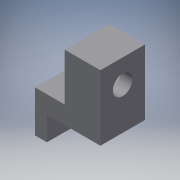
# Autodesk Inventor part: TMP_Holder_MTP
Saved by Autodesk Inventor 2019.4 (Build 234330000, 330)
## iProperties
Created: 2021-04-17
Part Number: TMP_Holder_MTP
Material: Generic
Document SubType Name: Modeling
Designer: diederichbenedict
Density: 1 g/cm^3
Appearance: Default
Author: diederichbenedict
Autodesk Inventor part; units mm, degrees
ref_plane "YZ Plane" through (0, 0, 0) normal (1, 0, 0) x (0, 1, 0)
ref_plane "XZ Plane" through (0, 0, 0) normal (0, 1, 0) x (-1, 0, 0)
ref_plane "XY Plane" through (0, 0, 0) normal (0, 0, 1) x (1, 0, 0)
sketch "Sketch1" plane through (0, 0, 0) normal (0, 0, 1) x (1, 0, 0)
  line L0 (31.7273, 1.5) -> (12.134, 1.5)
  line L1 (31.7273, -1.5) -> (12.134, -1.5)
  line L2 (16.2594, -4) -> (22.2594, -4)
  line L3 (22.2594, -4) -> (22.2594, 4)
  line L4 (22.2594, 4) -> (16.2594, 4)
  line L5 (16.2594, 4) -> (16.2594, -4)
  line L6 (16.2594, -4) -> (22.2594, 4) construction
  line L7 (22.2594, -4) -> (16.2594, 4) construction
  point P0 (0, 0)
  point P1 (19.2594, 0)
  dimension "d0" = 8
  dimension "d1" = 6
  constraints: 16 end point, 3 horizontal, 2 midpoint, 2 parallel, 1 perpendicular, 4 other
  measures "d0" distance between parallel lines of L2 L4
  measures "d1" distance between parallel lines of L3 L5
extrude "Extrusion1" add sketch "Sketch1" along normal mid plane 7.5
sketch "Sketch2" plane through (16.2594, -4, 3.75) normal (-1, 0, 0) x (0, 0, 1)
  line L0 (0, 0) -> (-7.5, 0) projected
  line L1 (0, 8) -> (0, 0) projected
  line L2 (-7.5, 8) -> (0, 8) projected
  line L3 (-7.5, 0) -> (-7.5, 8) projected
  circle A0 centre (-3.75, 4) radius 1.65
  dimension "d17" = 3.3
  constraints: 1 centre point
  measures "d17" diameter of A0
extrude "Extrusion2" cut sketch "Sketch2" against normal through all contours A0
sketch "Sketch3" plane through (16.2594, -4, 3.75) normal (-1, 0, 0) x (0, 0, 1)
  point P0 (-3.75, 4)
sketch "Sketch4" plane through (16.2594, -4, 3.75) normal (-1, 0, 0) x (0, 0, 1)
  line L0 (-0.953, 2.3546) -> (-3.803, 0.7091)
  line L1 (-3.803, 0.7091) -> (-6.653, 2.3546)
  line L2 (-6.653, 2.3546) -> (-6.653, 5.6454)
  line L3 (-6.653, 5.6454) -> (-3.803, 7.2909)
  line L4 (-3.803, 7.2909) -> (-0.953, 5.6454)
  line L5 (-0.953, 5.6454) -> (-0.953, 2.3546)
  line L6 (-7.5, 0) -> (-7.5, 8) projected
  point P0 (-3.803, 4)
  dimension "d18" = 5.7
  constraints: 12 end point, 1 parallel, 13 other
  measures "d18" distance between parallel lines of L0 L3
extrude "Extrusion3" cut sketch "Sketch4" against normal blind 4
sketch "Sketch5" plane through (0, 0, 3.75) normal (0, 0, 1) x (1, 0, 0)
  line L0 (16.2594, -4) -> (22.2594, -4) projected
  line L1 (22.2594, -4) -> (22.2594, 4) projected
  line L2 (22.2594, 4) -> (16.2594, 4) projected
  line L3 (16.2594, 4) -> (16.2594, -4) projected
  line L4 (16.2594, -4) -> (22.2594, -4) projected
  line L5 (22.2594, -4) -> (11.2594, -4)
  line L6 (11.2594, -4) -> (11.2594, -7)
  line L7 (11.2594, -7) -> (22.2594, -7)
  line L8 (22.2594, -7) -> (22.2594, -4)
  line L9 (11.2594, -7) -> (13.2594, -7)
  line L10 (13.2594, -7) -> (13.2594, -11)
  line L11 (13.2594, -11) -> (11.2594, -11)
  line L12 (11.2594, -11) -> (11.2594, -7)
  point P0 (0, 0)
  dimension "d13" = 11
  dimension "d14" = 3
  dimension "d15" = 2
  dimension "d16" = 4
  constraints: 16 end point, 4 parallel, 2 horizontal, 2 perpendicular
  measures "d13" distance of L7.end L6.end
  measures "d14" distance of L6.end L5.end
  measures "d15" distance of L10.end L11.end
  measures "d16" distance of L9.end L10.end
extrude "Extrusion4" add sketch "Sketch5" against normal up to surface (7.5 mm away) contours L0 L8 L7 L6 L5 | L7 L10 L11 L12
body "Solid1"
